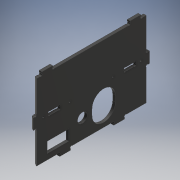
# Autodesk Inventor part: BA16
Saved by Autodesk Inventor 2017 (Build 210142000, 142)
## iProperties
Created: 2019-05-31
Part Number: BA16
Material: Polyethylene, High Density
Document SubType Name: Modeling
Designer: Dell
Density: 0.952 g/cm^3
Appearance: Smooth - Black
Mass: 274.487 g
Surface Area: 980.451 cm^2
Volume: 288.326 cm^3
Author: Dell
Autodesk Inventor part; units mm, degrees
ref_plane "YZ Plane" through (0, 0, 0) normal (1, 0, 0) x (0, 1, 0)
ref_plane "XZ Plane" through (0, 0, 0) normal (0, 1, 0) x (-1, 0, 0)
ref_plane "XY Plane" through (0, 0, 0) normal (0, 0, 1) x (1, 0, 0)
sketch "Sketch1" plane through (0, 0, 0) normal (0, 0, 1) x (1, 0, 0)
  line L0 (0, 0) -> (0, -195.6092) construction
  line L1 (0, -195.6092) -> (262.89, -347.3888) construction
  line L2 (262.89, -347.3888) -> (525.78, -195.6092) construction
  line L3 (525.78, -195.6092) -> (525.78, 0) construction
  line L4 (525.78, 0) -> (0, 0) construction
  line L5 (101.6, -254.268) -> (101.6, 0)
  line L6 (101.6, 0) -> (107.95, 0)
  line L7 (107.95, -257.9342) -> (101.6, -254.268)
  line L8 (107.95, 0) -> (107.95, -257.9342)
  point P0 (262.89, 0)
  dimension "d0" = 525.78
  dimension "d1" = 195.6092
  dimension "d2" = 120
  dimension "d3" = 6.35
  dimension "d4" = 101.6
  constraints: 18 end point, 4 point on line, 3 perpendicular, 1 collinear, 1 horizontal alignment, 1 midpoint, 1 parallel, 1 vertical, 1 vertical alignment
  measures "d0" distance of L3.end L0.start
  measures "d1" distance of L0.start L0.end
  measures "d2" angle of L2 L1
  measures "d3" distance between parallel lines of L5 L8
  measures "d4" distance between parallel lines of L0 L5
extrude "Extrusion1" add sketch "Sketch1" along normal blind 177.8
sketch "Sketch2" plane through (107.95, -257.9342, 0) normal (1, 0, 0) x (0, 0, -1)
  line L0 (0, 257.9342) -> (-177.8, 257.9342) projected
  line L1 (-101.6, 257.9342) -> (-76.2, 257.9342)
  line L2 (-76.2, 257.9342) -> (-76.2, 265.5542)
  line L3 (-76.2, 265.5542) -> (-101.6, 265.5542)
  line L4 (-101.6, 265.5542) -> (-101.6, 257.9342)
  line L5 (0, 3.6662) -> (-177.8, 3.6662) projected
  line L6 (-101.6, 3.6662) -> (-76.2, 3.6662)
  line L7 (-76.2, 3.6662) -> (-76.2, -7.62)
  line L8 (-76.2, -7.62) -> (-101.6, -7.62)
  line L9 (-101.6, -7.62) -> (-101.6, 3.6662)
  line L10 (0, 0) -> (-177.8, 0) projected
  point P0 (-88.9, 257.9342)
  point P1 (-88.9, 3.6662)
  dimension "d7" = 25.4
  dimension "d8" = 7.62
  dimension "d9" = 7.62
  constraints: 16 end point, 4 midpoint, 4 parallel, 2 horizontal, 2 perpendicular, 2 point on line, 1 vertical alignment
  measures "d7" distance of L3.end L2.end
  measures "d8" distance of L2.end L1.end
  measures "d9" distance between parallel lines of L8 L10
extrude "Extrusion2" add sketch "Sketch2" against normal blind 6.35
sketch "Sketch3" plane through (0, 0, 177.8) normal (0, 0, 1) x (1, 0, 0)
  line L0 (101.6, -254.268) -> (107.95, -257.9342) projected
  line L1 (107.95, -265.5542) -> (101.6, -265.5542) projected
  line L2 (107.95, -265.5542) -> (101.6, -261.888)
  line L3 (101.6, -265.5542) -> (101.6, -254.268) projected
  line L4 (101.6, -261.888) -> (101.6, -265.5542)
  point P0 (0, 0)
  constraints: 4 end point, 1 collinear, 1 parallel
extrude "Extrusion3" cut sketch "Sketch3" along normal through all both and the other way through all
sketch "Sketch4" plane through (101.6, -254.268, 0) normal (-1, 0, 0) x (0, 0, 1)
  line L0 (0, 203.468) -> (-7.62, 203.468)
  line L1 (-7.62, 203.468) -> (-7.62, 178.068)
  line L2 (-7.62, 178.068) -> (0, 178.068)
  line L3 (0, 178.068) -> (0, 203.468)
  line L4 (0, 0) -> (0, 254.268) projected
  line L5 (0, 76.468) -> (-7.62, 76.468)
  line L6 (-7.62, 76.468) -> (-7.62, 51.068)
  line L7 (-7.62, 51.068) -> (0, 51.068)
  line L8 (0, 51.068) -> (0, 76.468)
  line L9 (0, 254.268) -> (76.2, 254.268) projected
  dimension "d14" = 7.62
  dimension "d15" = 25.4
  dimension "d16" = 25.4
  dimension "d17" = 50.8
  dimension "d18" = 101.6
  constraints: 16 end point, 4 parallel, 2 horizontal, 2 perpendicular, 2 point on line, 1 vertical alignment
  measures "d14" distance of L0.start L0.end
  measures "d15" distance of L0.end L1.end
  measures "d16" distance of L5.end L6.end
  measures "d17" distance from line of L9 L0.end
  measures "d18" distance of L1.end L5.end
extrude "Extrusion4" add sketch "Sketch4" against normal blind 6.35
sketch "Sketch5" plane through (107.95, -257.9342, 177.8) normal (1, 0, 0) x (0, 0, -1)
  line L0 (165.1, 25.4) -> (139.7, 25.4)
  line L1 (139.7, 25.4) -> (139.7, 76.2)
  line L2 (139.7, 76.2) -> (165.1, 76.2)
  line L3 (165.1, 76.2) -> (165.1, 25.4)
  line L4 (177.8, 54.7342) -> (177.8, 0) projected
  line L5 (177.8, 0) -> (101.6, 0) projected
  point P0 (177.8, 257.9342)
  dimension "d21" = 25.4
  dimension "d22" = 50.8
  dimension "d23" = 12.7
  dimension "d24" = 25.4
  constraints: 8 end point, 2 parallel, 1 horizontal, 1 perpendicular
  measures "d21" distance of L1.end L2.end
  measures "d22" distance of L0.end L1.end
  measures "d23" distance between parallel lines of L4 L3
  measures "d24" distance between parallel lines of L5 L0
extrude "Extrusion5" cut sketch "Sketch5" against normal through all
sketch "Sketch6" plane through (101.6, -254.268, 177.8) normal (-1, 0, 0) x (0, 0, 1)
  line L0 (0, 254.268) -> (0, 0) projected
  line L1 (0, 241.568) -> (7.62, 241.568)
  line L2 (7.62, 241.568) -> (7.62, 216.168)
  line L3 (7.62, 216.168) -> (0, 216.168)
  line L4 (0, 216.168) -> (0, 241.568)
  line L5 (0, 34.4338) -> (7.62, 34.4338)
  line L6 (7.62, 34.4338) -> (7.62, 9.0338)
  line L7 (7.62, 9.0338) -> (0, 9.0338)
  line L8 (0, 9.0338) -> (0, 34.4338)
  line L9 (-76.2, 254.268) -> (0, 254.268) projected
  line L10 (-76.2, 0) -> (0, 0) projected
  point P0 (-177.8, 254.268)
  dimension "d27" = 7.62
  dimension "d28" = 25.4
  dimension "d29" = 25.4
  dimension "d30" = 12.7
  dimension "d34" = 181.7342
  constraints: 16 end point, 4 parallel, 2 horizontal, 2 perpendicular, 2 point on line, 1 vertical alignment
  measures "d27" distance of L2.end L3.end
  measures "d28" distance of L1.end L2.end
  measures "d29" distance of L5.end L6.end
  measures "d30" distance between parallel lines of L9 L1
  measures "d34" distance between parallel lines of L5 L3
extrude "Extrusion6" add sketch "Sketch6" against normal blind 6.35
sketch "Sketch7" plane through (101.6, -254.268, 101.6) normal (-1, 0, 0) x (0, 0, 1)
  line L0 (-6.35, 228.868) -> (-12.7, 228.868)
  line L1 (-12.7, 228.868) -> (-12.7, 203.468)
  line L2 (-12.7, 203.468) -> (-6.35, 203.468)
  line L3 (-6.35, 203.468) -> (-6.35, 228.868)
  line L4 (-6.35, 51.068) -> (-12.7, 51.068)
  line L5 (-12.7, 51.068) -> (-12.7, 25.668)
  line L6 (-12.7, 25.668) -> (-6.35, 25.668)
  line L7 (-6.35, 25.668) -> (-6.35, 51.068)
  line L8 (-6.35, 216.168) -> (-6.35, 38.368) construction
  line L9 (76.2, 216.168) -> (76.2, 34.4338) projected
  line L10 (-101.6, 203.468) -> (-101.6, 254.268) projected
  line L11 (0, 254.268) -> (76.2, 254.268) projected
  point P0 (-6.35, 127.268)
  point P1 (76.2, 125.3009)
  dimension "d35" = 6.35
  dimension "d36" = 25.4
  dimension "d37" = 6.35
  dimension "d38" = 25.4
  dimension "d39" = 177.8
  dimension "d40" = 88.9
  dimension "d43" = 25.4
  constraints: 18 end point, 4 midpoint, 4 parallel, 2 horizontal, 2 perpendicular, 1 point on line
  measures "d35" distance of L2.end L1.end
  measures "d36" distance of L1.end L0.end
  measures "d37" distance of L6.end L5.end
  measures "d38" distance of L5.end L4.end
  measures "d39" distance of L8.start L8.end
  measures "d40" distance between parallel lines of L10 L1
  measures "d43" distance from line of L11 L0.start
extrude "Extrusion7" cut sketch "Sketch7" against normal through all
sketch "Sketch8" plane through (101.6, -254.268, 101.6) normal (-1, 0, 0) x (0, 0, 1)
  circle A0 centre (-9.525, 176.1009) radius 2.25
  circle A1 centre (-9.525, 74.5009) radius 2.25
  line L0 (-9.525, 176.1009) -> (-9.525, 74.5009) construction
  line L1 (-6.35, 203.468) -> (-12.7, 203.468) projected
  line L2 (76.2, 216.168) -> (76.2, 34.4338) projected
  circle A2 centre (-9.525, 241.568) radius 2.25
  circle A3 centre (-9.525, 12.834) radius 2.25
  line L3 (-12.7, 228.868) -> (-6.35, 228.868) projected
  line L4 (-9.525, 228.868) -> (-9.525, 254.268) construction
  line L5 (-12.7, 25.668) -> (-6.35, 25.668) projected
  line L6 (-9.525, 25.668) -> (-9.525, 0) construction
  point P0 (-101.6, 254.268)
  point P1 (-9.525, 203.468)
  point P2 (-9.525, 125.3009)
  point P3 (76.2, 125.3009)
  point P4 (0, 254.268)
  point P5 (0, 0)
  dimension "d44" = 4.5
  dimension "d45" = 4.5
  dimension "d46" = 101.6
  dimension "d47" = 4.5
  dimension "d48" = 4.5
  constraints: 7 midpoint, 6 end point, 4 centre point, 3 horizontal alignment, 3 vertical, 2 coincident, 1 vertical alignment
  measures "d44" diameter of A0
  measures "d45" diameter of A1
  measures "d46" distance of L0.start L0.end
  measures "d47" diameter of A2
  measures "d48" diameter of A3
extrude "Extrusion8" cut sketch "Sketch8" against normal through all
sketch "Sketch9" plane through (107.95, 7.62, 101.6) normal (1, 0, 0) x (0, 0, -1)
  circle A0 centre (57.15, -157.5822) radius 11.5
  line L0 (101.6, -7.62) -> (25.4, -7.62) projected
  line L1 (101.6, -83.82) -> (101.6, -185.42) projected
  dimension "d51" = 23
  dimension "d52" = 149.9622
  dimension "d53" = 44.45
  constraints: 1 centre point
  measures "d51" diameter of A0
  measures "d52" distance from line of L0 A0.centre
  measures "d53" distance from line of L1 A0.centre
extrude "Extrusion9" cut sketch "Sketch9" against normal through all
sketch "Sketch10" plane through (107.95, 7.62, 101.6) normal (1, 0, 0) x (0, 0, -1)
  circle A0 centre (57.15, -157.5822) radius 11.5 construction
  circle A1 centre (9.525, -20.32) radius 2.25 construction
  circle A2 centre (9.525, -85.7871) radius 2.25 construction
  circle A3 centre (9.525, -187.3871) radius 2.25 construction
  circle A4 centre (9.525, -249.054) radius 2.25 construction
  line L0 (12.7, -33.02) -> (12.7, -58.42) construction
  line L1 (12.7, -58.42) -> (6.35, -58.42) construction
  line L2 (6.35, -58.42) -> (6.35, -33.02) construction
  line L3 (6.35, -33.02) -> (12.7, -33.02) construction
  line L4 (12.7, -210.82) -> (12.7, -236.22) construction
  line L5 (12.7, -236.22) -> (6.35, -236.22) construction
  line L6 (6.35, -236.22) -> (6.35, -210.82) construction
  line L7 (6.35, -210.82) -> (12.7, -210.82) construction
  line L8 (88.9, -189.3542) -> (88.9, -240.1542) construction
  line L9 (88.9, -240.1542) -> (63.5, -240.1542) construction
  line L10 (63.5, -240.1542) -> (63.5, -189.3542) construction
  line L11 (63.5, -189.3542) -> (88.9, -189.3542) construction
  line L12 (101.6, -265.5542) -> (25.4, -265.5542) construction
  line L13 (101.6, -210.82) -> (101.6, -265.5542) construction
  line L14 (101.6, -210.82) -> (109.22, -210.82) construction
  line L15 (109.22, -210.82) -> (109.22, -185.42) construction
  line L16 (109.22, -185.42) -> (101.6, -185.42) construction
  line L17 (101.6, -83.82) -> (101.6, -185.42) construction
  line L18 (101.6, -83.82) -> (109.22, -83.82) construction
  line L19 (109.22, -83.82) -> (109.22, -58.42) construction
  line L20 (109.22, -58.42) -> (101.6, -58.42) construction
  line L21 (101.6, -7.62) -> (101.6, -58.42) construction
  line L22 (101.6, -7.62) -> (25.4, -7.62) construction
  line L23 (25.4, -7.62) -> (25.4, 0) construction
  line L24 (25.4, 0) -> (0, 0) construction
  line L25 (0, 0) -> (0, -7.62) construction
  line L26 (0, -7.62) -> (-76.2, -7.62) construction
  line L27 (-76.2, -20.32) -> (-76.2, -7.62) construction
  line L28 (-76.2, -20.32) -> (-83.82, -20.32) construction
  line L29 (-83.82, -20.32) -> (-83.82, -45.72) construction
  line L30 (-83.82, -45.72) -> (-76.2, -45.72) construction
  line L31 (-76.2, -227.4542) -> (-76.2, -45.72) construction
  line L32 (-76.2, -227.4542) -> (-83.82, -227.4542) construction
  line L33 (-83.82, -227.4542) -> (-83.82, -252.8542) construction
  line L34 (-83.82, -252.8542) -> (-76.2, -252.8542) construction
  line L35 (-76.2, -265.5542) -> (-76.2, -252.8542) construction
  line L36 (0, -265.5542) -> (-76.2, -265.5542) construction
  line L37 (0, -265.5542) -> (0, -273.1742) construction
  line L38 (0, -273.1742) -> (25.4, -273.1742) construction
  line L39 (25.4, -273.1742) -> (25.4, -265.5542) construction
  line L40 (-78.4451, -47.9651) -> (-86.0651, -47.9651) construction
  line L41 (-86.0651, -47.9651) -> (-86.0651, -18.0749) construction
  line L42 (-86.0651, -18.0749) -> (-78.4451, -18.0749) construction
  line L43 (-78.4451, -18.0749) -> (-78.4451, -5.3749) construction
  line L44 (-78.4451, -5.3749) -> (-2.2451, -5.3749) construction
  line L45 (-2.2451, -5.3749) -> (-2.2451, 2.2451) construction
  line L46 (-2.2451, 2.2451) -> (27.6451, 2.2451) construction
  line L47 (27.6451, 2.2451) -> (27.6451, -5.3749) construction
  line L48 (27.6451, -5.3749) -> (103.8451, -5.3749) construction
  line L49 (103.8451, -5.3749) -> (103.8451, -56.1749) construction
  line L50 (103.8451, -56.1749) -> (111.4651, -56.1749) construction
  line L51 (111.4651, -56.1749) -> (111.4651, -86.0651) construction
  line L52 (111.4651, -86.0651) -> (103.8451, -86.0651) construction
  line L53 (103.8451, -86.0651) -> (103.8451, -183.1749) construction
  line L54 (103.8451, -183.1749) -> (111.4651, -183.1749) construction
  line L55 (111.4651, -183.1749) -> (111.4651, -213.0651) construction
  line L56 (111.4651, -213.0651) -> (103.8451, -213.0651) construction
  line L57 (103.8451, -213.0651) -> (103.8451, -267.7993) construction
  line L58 (103.8451, -267.7993) -> (27.6451, -267.7993) construction
  line L59 (27.6451, -267.7993) -> (27.6451, -275.4193) construction
  line L60 (27.6451, -275.4193) -> (-2.2451, -275.4193) construction
  line L61 (-2.2451, -275.4193) -> (-2.2451, -267.7993) construction
  line L62 (-2.2451, -267.7993) -> (-78.4451, -267.7993) construction
  line L63 (-78.4451, -267.7993) -> (-78.4451, -255.0993) construction
  line L64 (-78.4451, -255.0993) -> (-86.0651, -255.0993) construction
  line L65 (-86.0651, -255.0993) -> (-86.0651, -225.2091) construction
  line L66 (-86.0651, -225.2091) -> (-78.4451, -225.2091) construction
  line L67 (-78.4451, -225.2091) -> (-78.4451, -47.9651) construction
  line L68 (5.08, -237.49) -> (13.97, -237.49)
  line L69 (13.97, -237.49) -> (13.97, -209.55)
  line L70 (13.97, -209.55) -> (5.08, -209.55)
  line L71 (5.08, -209.55) -> (5.08, -237.49)
  line L72 (5.08, -59.69) -> (13.97, -59.69)
  line L73 (13.97, -59.69) -> (13.97, -31.75)
  line L74 (13.97, -31.75) -> (5.08, -31.75)
  line L75 (5.08, -31.75) -> (5.08, -59.69)
  line L76 (12.7, -58.42) -> (6.35, -58.42) projected
  circle A5 centre (-78.4451, -255.0993) radius 3.175
  circle A6 centre (-78.4451, -225.2091) radius 3.175
  line L77 (-76.2, -45.72) -> (-76.2, -227.4542) projected
  circle A7 centre (-78.4451, -47.9651) radius 3.175
  circle A8 centre (-78.4451, -18.0749) radius 3.175
  line L78 (0, -7.62) -> (-76.2, -7.62) projected
  circle A9 centre (-2.2451, -5.3749) radius 3.175
  circle A10 centre (27.6451, -5.3749) radius 3.175
  circle A11 centre (103.8451, -56.1749) radius 3.175
  circle A12 centre (103.8451, -86.0651) radius 3.175
  line L79 (101.6, -185.42) -> (101.6, -83.82) projected
  circle A13 centre (103.8451, -183.1749) radius 3.175
  line L80 (109.22, -210.82) -> (101.6, -210.82) projected
  circle A14 centre (103.8451, -213.0651) radius 3.175
  line L81 (0, -265.5542) -> (-76.2, -265.5542) projected
  circle A15 centre (-2.2451, -267.7993) radius 3.175
  circle A16 centre (27.6451, -267.7993) radius 3.175
  line L82 (7.3251, -235.2449) -> (11.7249, -235.2449)
  line L83 (11.7249, -235.2449) -> (11.7249, -211.7951)
  line L84 (11.7249, -211.7951) -> (7.3251, -211.7951)
  line L85 (7.3251, -211.7951) -> (7.3251, -235.2449)
  circle A17 centre (7.3251, -235.2449) radius 3.175
  circle A18 centre (7.3251, -211.7951) radius 3.175
  circle A19 centre (11.7249, -211.7951) radius 3.175
  circle A20 centre (11.7249, -235.2449) radius 3.175
  line L86 (7.3251, -57.4449) -> (11.7249, -57.4449)
  line L87 (11.7249, -57.4449) -> (11.7249, -33.9951)
  line L88 (11.7249, -33.9951) -> (7.3251, -33.9951)
  line L89 (7.3251, -33.9951) -> (7.3251, -57.4449)
  circle A21 centre (7.3251, -57.4449) radius 3.175
  circle A22 centre (11.7249, -57.4449) radius 3.175
  circle A23 centre (11.7249, -33.9951) radius 3.175
  circle A24 centre (7.3251, -33.9951) radius 3.175
  point P0 (101.6, -7.62)
  point P1 (9.525, -236.22)
  point P2 (9.525, -237.49)
  point P3 (9.525, -58.42)
  point P4 (9.525, -59.69)
  point P5 (9.525, -58.42)
  point P6 (6.35, -223.52)
  point P7 (5.08, -223.52)
  point P8 (6.35, -45.72)
  point P9 (5.08, -45.72)
  dimension "d59" = 6.35
  dimension "d60" = 6.35
  dimension "d61" = 6.35
  dimension "d56" = 1.27
  dimension "d57" = 1.27
  dimension "d58" = 1.27
  constraints: 88 end point, 20 coincident, 9 midpoint, 8 parallel, 4 perpendicular, 2 horizontal, 2 horizontal alignment, 2 vertical alignment, 1 point on line, 93 other
  measures "d56" distance between parallel lines of L71 L6
  measures "d57" distance between parallel lines of L68 L5
  measures "d58" distance between parallel lines of L72 L1
extrude "Extrusion10" cut sketch "Sketch10" against normal through all
sketch "Sketch11" plane through (107.95, 7.62, 101.6) normal (1, 0, 0) x (0, 0, -1)
  circle A0 centre (64.15, -107.5822) radius 27.5
  circle A1 centre (57.15, -157.5822) radius 11.5 projected
  circle A2 centre (50.15, -107.5822) radius 27.5
  line L0 (50.15, -135.0822) -> (64.15, -135.0822)
  line L1 (50.15, -80.0822) -> (64.15, -80.0822)
  point P0 (101.6, -7.62)
  dimension "d64" = 55
  dimension "d65" = 7
  dimension "d66" = 50
  dimension "d69" = 55
  dimension "d70" = 7
  constraints: 4 end point, 4 point on circle, 4 tangent, 2 centre point, 1 horizontal alignment
  measures "d64" diameter of A0
  measures "d65" horizontal distance of A0.centre A1.centre
  measures "d66" vertical distance of A1.centre A0.centre
  measures "d69" diameter of A2
  measures "d70" horizontal distance of A2.centre A1.centre
extrude "Extrusion11" cut sketch "Sketch11" against normal through all contours A0 A2 | A0 A2 L1 | L0 A2 A0 | A2 A0 | A0 A2
equation "\"d3\" = Panel_Thickness"
equation "\"d8\" = Panel_Thickness + Fit_Tolerance"
equation "\"d9\" = Panel_Thickness + Fit_Tolerance"
equation "\"d10\" = Panel_Thickness"
equation "\"d14\" = Panel_Thickness + Fit_Tolerance"
equation "\"d19\" = Panel_Thickness"
equation "\"d25\" = Panel_Thickness"
equation "\"d27\" = Panel_Thickness + Fit_Tolerance"
equation "\"d32\" = Panel_Thickness"
equation "\"d35\" = Panel_Thickness"
equation "\"d37\" = Panel_Thickness"
equation "\"d41\" = Panel_Thickness"
equation "\"d49\" = Panel_Thickness"
equation "\"d54\" = Panel_Thickness"
equation "\"d59\" = Tool_Dia"
equation "\"d60\" = Tool_Dia"
equation "\"d61\" = Tool_Dia"
equation "\"d56\" = Fit_Tolerance"
equation "\"d57\" = Fit_Tolerance"
equation "\"d58\" = Fit_Tolerance"
equation "\"d62\" = Panel_Thickness"
equation "\"Panel_Thickness\" = 6.35"
equation "\"Fit_Tolerance\" = 1.27"
equation "\"Tool_Dia\" = 6.35"
body "Solid1"
